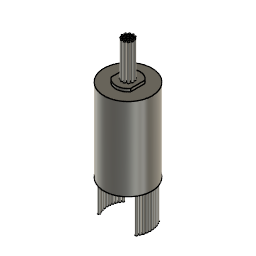
slip_ring_6.75Rx23.2Lmm_v1 (Autodesk Fusion 360 design; units mm, degrees)
Autodesk Fusion 360 part; units mm, degrees
sketch "Sketch1" plane through (0, 0, 0) normal (0, 0, 1) x (1, 0, 0)
sketch "Sketch2" plane through (0, 0, 0) normal (0, 0, 1) x (1, 0, 0)
  circle A0 centre (0, 0) radius 6.75
  dimension "d1" = 13.5
  constraint coincident A0.centre origin
  measures "d1" diameter of A0
extrude "Extrude1" add sketch "Sketch2" along normal blind 23.2
sketch "Sketch3" plane through (0, 0, 23.2) normal (0, 0, 1) x (-1, 0, 0)
  circle A0 centre (0, 0) radius 6.75
  line L0 (-2.75, -1.9994) -> (-2.75, 1.9994)
  line L1 (2.75, 1.9994) -> (2.75, -1.9994)
  arc A1 (2.75, 1.9994) -> (-2.75, 1.9994) centre (0, 0) ccw
  arc A2 (-2.75, -1.9994) -> (2.75, -1.9994) centre (0, 0) ccw
  dimension "d4" = 6.8
  constraint coincident A0.centre A1.centre
  constraint vertical L0
  constraint vertical L1
  constraint concentric A1 A2
  measures "d4" diameter of A1
extrude "Extrude2" add sketch "Sketch3" along normal blind 0.8 contours L0 L1 A1 A2
sketch "Sketch5" plane through (0, 0, 24) normal (0, 0, 1) x (-1, 0, 0)
  arc A0 (2.75, 1.9994) -> (-2.75, 1.9994) centre (0, 0) ccw
  line L0 (-2.75, 1.9994) -> (-2.75, -1.9994)
  arc A1 (-2.75, -1.9994) -> (2.75, -1.9994) centre (0, 0) ccw
  line L1 (2.75, -1.9994) -> (2.75, 1.9994)
  circle A2 centre (0, 0) radius 0.3
  circle A3 centre (0, -0.7865) radius 0.3
  circle A4 centre (0.5561, -0.5561) radius 0.3
  circle A5 centre (0.7865, 0) radius 0.3
  circle A6 centre (0.5561, 0.5561) radius 0.3
  circle A7 centre (0, 0.7865) radius 0.3
  circle A8 centre (-0.5561, 0.5561) radius 0.3
  circle A9 centre (-0.7865, 0) radius 0.3
  circle A10 centre (-0.5561, -0.5561) radius 0.3
  circle A11 centre (0.007, -1.4) radius 0.3
  circle A12 centre (0.7628, -1.174) radius 0.3
  circle A13 centre (1.2764, -0.5752) radius 0.3
  circle A14 centre (1.3848, 0.2061) radius 0.3
  circle A15 centre (1.0535, 0.9221) radius 0.3
  circle A16 centre (0.3877, 1.3453) radius 0.3
  circle A17 centre (-0.4011, 1.3413) radius 0.3
  circle A18 centre (-1.0626, 0.9115) radius 0.3
  circle A19 centre (-1.3867, 0.1923) radius 0.3
  circle A20 centre (-1.2706, -0.5879) radius 0.3
  circle A21 centre (-0.751, -1.1815) radius 0.3
  dimension "d18" = 0.6
  dimension "d19" = 0.6
  dimension "d21" = 360
  dimension "d22" = 0.6
  dimension "d23" = 0.7865
  dimension "d24" = 1.4
  dimension "d26" = 360
  constraint coincident A0.centre A1.centre
  measures "d18" diameter of A2
  measures "d19" diameter of A3
  measures "d22" diameter of A11
  measures "d23" distance of A0.centre A3.centre
  measures "d24" vertical distance of A0.centre A11.centre
extrude "Extrude4" add sketch "Sketch5" along normal blind 10 contours A2 | A3 | A4 | A10 | A5 | A9 | A6 | A8 | A7 | A11 | A12 | A13 | A14 | A15 | A16 | A17 | A18 | A19 | A20 | A21
sketch "Sketch6" plane through (0, 0, 0) normal (0, 0, -1) x (1, 0, 0)
  circle A0 centre (0, 0) radius 6.75
  circle A1 centre (0, 0) radius 5.25
  circle A2 centre (0, 0) radius 6 construction
  circle A3 centre (-6, 0) radius 0.35
  circle A4 centre (-5.9527, -0.752) radius 0.35
  circle A5 centre (-5.8115, -1.4921) radius 0.35
  circle A6 centre (-5.5787, -2.2087) radius 0.35
  circle A7 centre (-5.2578, -2.8905) radius 0.35
  circle A8 centre (-4.8541, -3.5267) radius 0.35
  circle A9 centre (4.8541, -3.5267) radius 0.35
  circle A10 centre (5.2578, -2.8905) radius 0.35
  circle A11 centre (5.5787, -2.2087) radius 0.35
  circle A12 centre (5.8115, -1.4921) radius 0.35
  circle A13 centre (5.9527, -0.752) radius 0.35
  circle A14 centre (6, 0) radius 0.35
  circle A15 centre (5.9527, 0.752) radius 0.35
  circle A16 centre (5.8115, 1.4921) radius 0.35
  circle A17 centre (5.5787, 2.2087) radius 0.35
  circle A18 centre (5.2578, 2.8905) radius 0.35
  circle A19 centre (-5.2578, 2.8905) radius 0.35
  circle A20 centre (-5.5787, 2.2087) radius 0.35
  circle A21 centre (-5.8115, 1.4921) radius 0.35
  circle A22 centre (-5.9527, 0.752) radius 0.35
  dimension "d29" = 10.5
  dimension "d30" = 12
  dimension "d31" = 0.7
  dimension "d33" = 360
  constraint concentric A0 A1
  constraint concentric A1 A2
  constraint coincident A2 A3.centre
  measures "d29" diameter of A1
  measures "d30" diameter of A2
  measures "d31" diameter of A3
extrude "Extrude5" add sketch "Sketch6" along normal blind 10 contours A3 | A4 | A5 | A6 | A7 | A8 | A9 | A10 | A11 | A12 | A13 | A14 | A15 | A16 | A17 | A18 | A19 | A20 | A21 | A22
